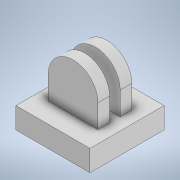
# Autodesk Inventor part: Soporte
Saved by Autodesk Inventor 2021 (Build 250183000, 183)
## iProperties
Created: 2022-01-12
Part Number: Soporte
Material: Generic
Document SubType Name: Modeling
Designer: Yeison
Density: 1 g/cm^3
Appearance: Default
Author: Yeison
Autodesk Inventor part; units mm, degrees
ref_plane "YZ Plane" through (0, 0, 0) normal (1, 0, 0) x (0, 1, 0)
ref_plane "XZ Plane" through (0, 0, 0) normal (0, 1, 0) x (-1, 0, 0)
ref_plane "XY Plane" through (0, 0, 0) normal (0, 0, 1) x (1, 0, 0)
sketch "Sketch1" plane through (0, 0, 0) normal (0, 0, 1) x (1, 0, 0)
  circle A0 centre (0, 0) radius 5.5
  line L0 (5.5, 0) -> (23.5, 0)
  line L1 (-5.5, 0) -> (-23.5, 0)
  arc A1 (23.5, 0) -> (-23.5, 0) centre (0, 0) ccw
  line L2 (-23.5, 0) -> (-23.5, -22)
  line L3 (-23.5, 0) -> (-1.5, 0) construction
  line L4 (-23.5, -22) -> (23.5, -22)
  line L5 (23.5, -22) -> (23.5, 0)
  dimension "d0" = 11
  dimension "d1" = 18
  dimension "d2" = 18
  dimension "d3" = 22
  dimension "d4" = 90
  constraints: 12 end point, 4 point on circle, 3 horizontal, 3 perpendicular, 2 centre point, 2 coincident, 1 point on line, 1 vertical
  measures "d0" diameter of A0
  measures "d1" distance of L0.start L0.end
  measures "d2" distance of L1.start L1.end
  measures "d3" distance of L2.start L2.end
  measures "d4" angle of L2 L3
extrude "Extrusion1" add sketch "Sketch1" along normal blind 10 and the other way blind 1 contours L0 L5 L4 L2 L1 A0 | A0 L1 A1 L0
sketch "Sketch2" plane through (0, 0, -1) normal (0, 0, -1) x (-1, 0, 0)
  circle A0 centre (0, 0) radius 5.5
  constraints: 1 centre point, 1 coincident
extrude "Extrusion2" add sketch "Sketch2" against normal blind 1
ref_plane "Work Plane1" through (0, 0, 15) normal (0, 0, 1) x (1, 0, 0)
mirror "Mirror1" about plane through (0, 0, 15) normal (0, 0, 1) of "Extrusion1", "Extrusion2"
ref_plane "Work Plane2" through (-23.5, -22, 10) normal (0, -1, 0) x (1, 0, 0)
sketch "Sketch3" plane through (-23.5, -22, 10) normal (0, -1, 0) x (1, 0, 0)
  line L0 (47, 21) -> (47, 10) projected
  line L1 (47, -11) -> (47, 0) projected
  line L2 (47, 21) -> (47, -11)
  line L3 (0, -11) -> (0, 0) projected
  line L4 (47, -11) -> (0, -11)
  line L5 (0, 21) -> (0, 10) projected
  line L6 (0, -11) -> (0, 21)
  line L7 (0, 21) -> (47, 21)
  line L8 (-11.5, -30) -> (58.5, -30)
  line L9 (58.5, -30) -> (58.5, 40)
  line L10 (58.5, 40) -> (-11.5, 40)
  line L11 (-11.5, 40) -> (-11.5, -30)
  line L12 (-11.5, -30) -> (58.5, 40) construction
  line L13 (58.5, -30) -> (-11.5, 40) construction
  point P0 (23.5, -10)
  point P1 (23.5, 5)
  dimension "d13" = 70
  dimension "d14" = 70
  constraints: 20 end point, 4 perpendicular, 2 midpoint, 2 parallel, 1 horizontal, 1 vertical
  measures "d13" distance of L10.end L9.end
  measures "d14" distance of L9.end L8.end
extrude "Extrusion3" add sketch "Sketch3" along normal blind 20 contours L0 L2 L1 L4 L3 L6 L5 L7 | L11 L10 L9 L8
body "Solid1"
